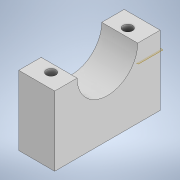
# Autodesk Inventor part: motor_mount_UP
Saved by Autodesk Inventor 2020 (Build 240168000, 168)
## iProperties
Created: 2024-09-09
Part Number: motor_mount_UP
Material: Типовые
Document SubType Name: Modeling
Designer: Ivan
Density: 1 g/cm^3
Appearance: По умолчанию
Author: Ivan
Autodesk Inventor part; units mm, degrees
ref_plane "YZ Plane" through (0, 0, 0) normal (1, 0, 0) x (0, 1, 0)
ref_plane "XZ Plane" through (0, 0, 0) normal (0, 1, 0) x (-1, 0, 0)
ref_plane "XY Plane" through (0, 0, 0) normal (0, 0, 1) x (1, 0, 0)
sketch "Эскиз1" plane through (0, 0, 0) normal (0, 1, 0) x (-1, 0, 0)
  line L0 (7.5, 22) -> (-7.5, 22)
  line L1 (-7.5, 22) -> (-7.5, -22)
  line L2 (-7.5, -22) -> (7.5, -22)
  line L3 (7.5, -22) -> (7.5, 22)
  line L4 (-7.5, 22) -> (7.5, -22) construction
  line L5 (0, 22) -> (0, -22) construction
  circle A0 centre (0, 16) radius 2
  line L6 (7.5, 0) -> (-7.5, 0) construction
  circle A1 centre (0, -16) radius 2
  point P0 (0, 0)
  point P1 (0, 0)
  dimension "d0" = 15
  dimension "d1" = 44
  dimension "d2" = 16
  dimension "d3" = 4
  constraints: 14 end point, 5 midpoint, 2 centre point, 2 coincident, 2 parallel, 1 horizontal, 1 perpendicular, 1 point on line, 1 symmetric about line, 1 other
  measures "d0" distance of L2.end L1.end
  measures "d1" distance of L0.end L1.end
  measures "d2" distance of point (0, 0) point (0, 16)
  measures "d3" diameter of A0
extrude "Выдавливание1" add sketch "Эскиз1" along normal blind 29
sketch "Эскиз2" plane through (7.5, 0, 22) normal (1, 0, 0) x (0, 0, -1)
  line L0 (0, 29) -> (44, 29) projected
  circle A0 centre (22, 29) radius 12.65
  point P0 (22, 0)
  dimension "d6" = 25.3
  constraints: 1 centre point, 1 midpoint
  measures "d6" diameter of A0
extrude "Выдавливание2" cut sketch "Эскиз2" against normal through all
ref_plane "РабПлоскость1" through (0, 22, 0) normal (0, 1, 0) x (1, 0, 0)
sketch "Эскиз3" plane through (0, 22, 0) normal (0, 1, 0) x (1, 0, 0)
  circle A0 centre (0, 16) radius 2 projected
  circle A1 centre (0, -16) radius 2 projected
  point P0 (0, 0)
extrude "Выдавливание3" add sketch "Эскиз3" against normal blind 15
